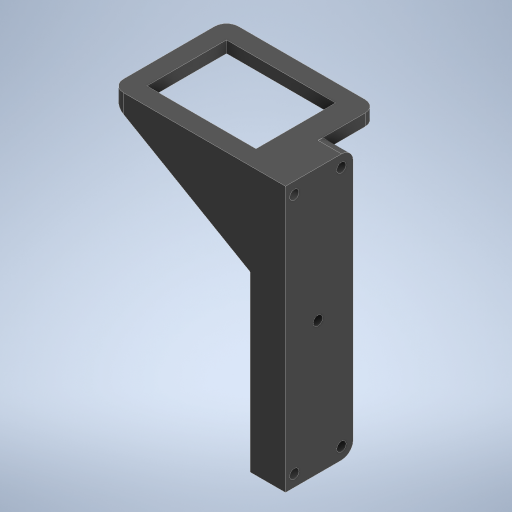
# Autodesk Inventor part: button_setter
Saved by Autodesk Inventor 2024.1 (Build 281209000, 209)
## iProperties
Created: 2024-02-15
Part Number: button_setter
Material: 一般
Document SubType Name: Modeling
Designer: hibik
Density: 1 g/cm^3
Appearance: 既定
Author: hibik
Autodesk Inventor part; units mm, degrees
ref_plane "YZ Plane" through (0, 0, 0) normal (1, 0, 0) x (0, 1, 0)
ref_plane "XZ Plane" through (0, 0, 0) normal (0, 1, 0) x (-1, 0, 0)
ref_plane "XY Plane" through (0, 0, 0) normal (0, 0, 1) x (1, 0, 0)
sketch "スケッチ1" plane through (0, 0, 0) normal (1, 0, 0) x (0, 1, 0)
  line L0 (45, 0) -> (0, 0)
  line L1 (0, 0) -> (0, -11.5)
  line L2 (0, -11.5) -> (45, -11.5)
  line L3 (45, -11.5) -> (45, 0)
  dimension "d0" = 45
  dimension "d1" = 11.5
  constraints: 8 end point, 2 parallel, 1 coincident, 1 horizontal, 1 perpendicular
  measures "d0" distance of L0.start L0.end
  measures "d1" distance of L2.end L0.start
extrude "押し出し1" add sketch "スケッチ1" along normal blind 3
sketch "スケッチ2" plane through (3, 0, 0) normal (1, 0, 0) x (0, 0, -1)
  circle A0 centre (1.5, 43) radius 0.8 projected
  circle A1 centre (9.4807, 43) radius 0.8 projected
  circle A2 centre (9.5, 2) radius 0.8 projected
  circle A3 centre (1.5, 2) radius 0.8 projected
  circle A4 centre (5.5, 22.5) radius 0.8 projected
  point P0 (0, 0)
extrude "押し出し2" cut sketch "スケッチ2" against normal through all
fillet "フィレット1" radius 2 2 edges at (1.5, 45, -11.5) (1.5, 0, -11.5)
sketch "スケッチ5" plane through (0, 45, 0) normal (0, 1, 0) x (1, 0, 0)
  line L0 (-5, 3) -> (-23.5, 3)
  line L1 (-23.5, 3) -> (-23.5, 16.5)
  line L2 (-23.5, 16.5) -> (-5, 16.5)
  line L3 (-5, 16.5) -> (-5, 3)
  line L4 (0, 0) -> (-26.5, 0)
  line L5 (-26.5, 0) -> (-26.5, 19.5)
  line L6 (-26.5, 19.5) -> (0, 19.5)
  line L7 (0, 19.5) -> (0, 0)
  point P0 (3, 0)
  dimension "d15" = 18.5
  dimension "d16" = 13.5
  dimension "d17" = 3
  dimension "d18" = 5
  dimension "d19" = 3
  dimension "d20" = 3
  constraints: 16 end point, 4 parallel, 2 horizontal, 2 perpendicular, 1 coincident
  measures "d15" distance of L1.end L2.end
  measures "d16" distance of L0.end L1.end
  measures "d17" distance between parallel lines of L4 L0
  measures "d18" distance between parallel lines of L7 L3
  measures "d19" distance between parallel lines of L5 L1
  measures "d20" distance between parallel lines of L6 L2
extrude "押し出し4" add sketch "スケッチ5" against normal blind 2
sketch "スケッチ6" plane through (0, 0, 0) normal (0, 0, 1) x (1, 0, 0)
  line L0 (0, 43) -> (-26.5, 43) projected
  line L1 (-26.5, 43) -> (0, 27.7002)
  line L2 (0, 25.5) -> (0, 40) projected
  line L3 (0, 43) -> (0, 0) projected
  dimension "d23" = 30
  constraints: 2 end point, 1 point on line
  measures "d23" angle of L0 L1
extrude "押し出し5" add sketch "スケッチ6" against normal up to surface (3 mm away)
sketch "スケッチ7" plane through (0, 45, -9.5) normal (1, 0, 0) x (0, 0, -1)
  line L0 (0, 0) -> (10, 0) projected
  arc A0 (2, -2) -> (0, 0) centre (0, -2) ccw projected
  line L1 (10, -2) -> (2, -2) projected
  line L2 (10, 0) -> (10, -2) projected
  line L3 (0, 0) -> (10, 0) projected
  point P0 (-9.5, -45)
extrude "押し出し6" cut sketch "スケッチ7" against normal blind 1
fillet "フィレット2" radius 2 3 edges at (-26.5, 44, 0) (-26.5, 44, -19.5) (-1, 44, -19.5)
sketch "スケッチ8" plane through (0, 0, 0) normal (-1, 0, 0) x (0, 0, 1)
  circle A0 centre (-1.5, 2) radius 0.8 projected
  circle A1 centre (-9.5, 2) radius 0.8 projected
  circle A2 centre (-5.5, 22.5) radius 0.8 projected
  line L0 (0, 27.7002) -> (-3, 27.7002) projected
  line L1 (-3, 27.7002) -> (-3, 43) projected
  line L2 (-3, 43) -> (-8.6807, 43) projected
  arc A3 (-10.2807, 43) -> (-8.6807, 43) centre (-9.4807, 43) ccw projected
  line L3 (-10.2807, 43) -> (-11.5, 43) projected
  line L4 (-11.5, 2) -> (-11.5, 43) projected
  arc A4 (-11.5, 2) -> (-9.5, 0) centre (-9.5, 2) ccw projected
  line L5 (0, 0) -> (-9.5, 0) projected
  line L6 (0, 27.7002) -> (0, 0) projected
  line L7 (-3, 39.3409) -> (0, 39.3409)
  line L8 (0, 39.3409) -> (0, 27.7002)
  line L9 (0, 27.7002) -> (-3, 27.7002)
  line L10 (-3, 27.7002) -> (-3, 39.3409)
  constraints: 8 end point, 2 parallel, 1 horizontal, 1 perpendicular, 1 point on line
extrude "押し出し7" add sketch "スケッチ8" along normal blind 3
equation "\"d19\" = d17"
equation "\"d20\" = d17"
